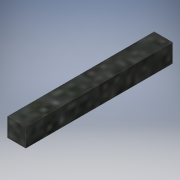
# Autodesk Inventor part: .125in. X .125in. Key, 1in. Long
Saved by Autodesk Inventor 2019 (Build 230136000, 136)
## iProperties
Created: 2018-11-13
Part Number: .125in. X .125in. Key, 1in. Long
Material: Steel
Document SubType Name: Modeling
Designer: Alex Barnett
Density: 7.85 g/cm^3
Appearance: Plate
Author: Alex Barnett
Autodesk Inventor part; units mm, degrees
ref_plane "YZ Plane" through (0, 0, 0) normal (1, 0, 0) x (0, 1, 0)
ref_plane "XZ Plane" through (0, 0, 0) normal (0, 1, 0) x (-1, 0, 0)
ref_plane "XY Plane" through (0, 0, 0) normal (0, 0, 1) x (1, 0, 0)
sketch "Sketch1" plane through (0, 0, 0) normal (0, 0, 1) x (1, 0, 0)
  line L0 (-1.5875, -1.5875) -> (1.5875, -1.5875)
  line L1 (1.5875, -1.5875) -> (1.5875, 1.5875)
  line L2 (1.5875, 1.5875) -> (-1.5875, 1.5875)
  line L3 (-1.5875, 1.5875) -> (-1.5875, -1.5875)
  line L4 (-1.5875, -1.5875) -> (1.5875, 1.5875) construction
  line L5 (1.5875, -1.5875) -> (-1.5875, 1.5875) construction
  point P0 (0, 0)
  dimension "d0" = 3.175
  dimension "d1" = 3.175
  constraints: 12 end point, 2 midpoint, 2 parallel, 1 horizontal, 1 perpendicular
  measures "d0" distance of L2.end L1.end
  measures "d1" distance of L1.end L0.end
extrude "Extrusion1" add sketch "Sketch1" along normal mid plane 25.4
body "Solid1"
